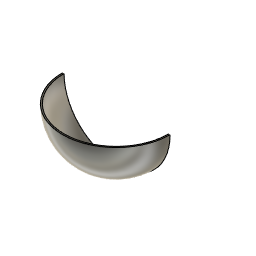
Adam Funnel v8 (Autodesk Fusion 360 design; units mm, degrees)
Autodesk Fusion 360 part; units mm, degrees
sketch "Sketch1" plane through (0, 0, 0) normal (0, 0, 1) x (1, 0, 0)
  line L0 (0, 0) -> (0, -38.1)
  arc A0 (0, -38.1) -> (38.1, 0) centre (0, 0) ccw
  arc A1 (-38.1, 0) -> (0, -38.1) centre (0, 0) ccw
  arc A2 (38.1, 0) -> (24.6636, 43.2107) centre (-38.1, 0) ccw
  arc A3 (-24.6636, 43.2107) -> (-38.1, 0) centre (38.1, 0) ccw
  line L1 (0, 58.6695) -> (0, -38.1)
  arc A4 (24.6636, 43.2107) -> (-24.6636, 43.2107) centre (0, 22.2311) ccw
  dimension "d1" = 38.1
  constraint coincident L0.start A0.centre
  constraint vertical L0
  constraint coincident A1.start A2.centre
  constraint coincident A0.end A2.start
  constraint horizontal A2.end A3.start
  constraint parallel L0 L1
  measures "d1" distance of L0.start L0.end
revolve "Revolve1" add sketch "Sketch1" angle 180 about axis through (0, 58.6695, 0) along (0, 1, 0) contours L0 A0 A2 L1 A4
shell "Shell2" thickness 1 removed faces 2 at (25.2155, 3.0555, 0) at (-25.2155, 3.0555, 0)
move_body "Move1" bodies 1 to x (1, 0, 0) y (0, 1, 0) z (0, 0, 1) at (0, 0, 90)
